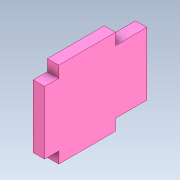
# Autodesk Inventor part: SideWall
Saved by Autodesk Inventor 2021 (Build 250183000, 183)
## iProperties
Created: 2021-08-31
Part Number: SideWall
Material: ABS Plastic
Document SubType Name: Modeling
Designer: digge
Density: 1.06 g/cm^3
Appearance: Pink
Author: digge
Autodesk Inventor part; units mm, degrees
ref_plane "YZ Plane" through (0, 0, 0) normal (1, 0, 0) x (0, 1, 0)
ref_plane "XZ Plane" through (0, 0, 0) normal (0, 1, 0) x (-1, 0, 0)
ref_plane "XY Plane" through (0, 0, 0) normal (0, 0, 1) x (1, 0, 0)
sketch "Sketch1" plane through (0, 0, 0) normal (1, 0, 0) x (0, 1, 0)
  line L0 (69.0933, 8.2135) -> (13.6933, 8.2135)
  line L1 (13.6933, 8.2135) -> (13.6933, 35.7135)
  line L2 (13.6933, 35.7135) -> (3.6933, 35.7135)
  line L3 (3.6933, 35.7135) -> (3.6933, 85.7135)
  line L4 (3.6933, 85.7135) -> (13.6933, 85.7135)
  line L5 (13.6933, 85.7135) -> (13.6933, 98.2135)
  line L6 (13.6933, 98.2135) -> (69.0933, 98.2135)
  line L7 (69.0933, 98.2135) -> (69.0933, 85.7135)
  line L8 (69.0933, 85.7135) -> (79.0933, 85.7135)
  line L9 (79.0933, 85.7135) -> (79.0933, 35.7135)
  line L10 (79.0933, 35.7135) -> (69.0933, 35.7135)
  line L11 (69.0933, 35.7135) -> (69.0933, 8.2135)
  point P0 (0, 0)
  dimension "d0" = 55.4
  dimension "d1" = 10
  dimension "d2" = 10
  dimension "d3" = 10
  dimension "d4" = 27.5
  dimension "d5" = 12.5
  dimension "d8" = 50
  constraints: 24 end point, 8 perpendicular, 3 point on line, 2 horizontal, 1 parallel, 1 vertical
  measures "d0" distance of L5.end L6.end
  measures "d1" distance of L7.end L8.end
  measures "d2" distance of L3.end L4.end
  measures "d3" distance of L1.end L2.end
  measures "d4" distance of L10.end L0.start
  measures "d5" distance of L6.end L7.end
  measures "d8" distance of L8.end L9.end
extrude "Extrusion1" add sketch "Sketch1" along normal blind 10
equation "\"d1\" = Width"
equation "\"d2\" = Width"
equation "\"d3\" = Width"
equation "\"d6\" = Width"
equation "\"Width\" = 10"
body "Solid1"
